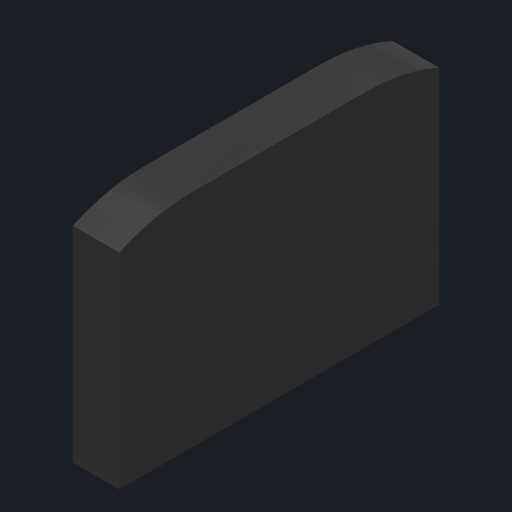
# Autodesk Inventor part: CARCASA_PANTALLA
Saved by Autodesk Inventor 2024.3 (Build 283343000, 343)
## iProperties
Created: 2024-07-02
Part Number: CARCASA_PANTALLA
Material: Steel, Mild, Welded
Document SubType Name: Modeling
Designer: Niler
Density: 7.85 g/cm^3
Appearance: Weld - Steel Mild
Author: Niler
Autodesk Inventor part; units mm, degrees
ref_plane "YZ Plane" through (0, 0, 0) normal (1, 0, 0) x (0, 1, 0)
ref_plane "XZ Plane" through (0, 0, 0) normal (0, 1, 0) x (-1, 0, 0)
ref_plane "XY Plane" through (0, 0, 0) normal (0, 0, 1) x (1, 0, 0)
sketch "Sketch1" plane through (0, 0, 0) normal (1, 0, 0) x (0, 1, 0)
  line L0 (-190, 275) -> (190, 275)
  line L1 (190, 275) -> (190, -275)
  line L2 (190, -275) -> (-190, -275)
  line L3 (-190, -275) -> (-190, 275)
  line L4 (-190, 275) -> (190, -275) construction
  line L5 (190, 275) -> (-190, -275) construction
  point P0 (0, 0)
  dimension "d0" = 550
  dimension "d1" = 380
  constraints: 12 end point, 2 midpoint, 2 parallel, 1 horizontal, 1 perpendicular
  measures "d0" distance of L0.end L1.end
  measures "d1" distance of L1.end L2.end
extrude "Extrusion1" add sketch "Sketch1" along normal mid plane 80
sketch "Sketch2" plane through (40, 0, 0) normal (1, 0, 0) x (0, 0, -1)
  line L0 (275, -190) -> (275, 190) projected
  line L1 (275, 190) -> (-275, 190) projected
  line L2 (-275, 190) -> (-275, -190) projected
  line L3 (-275, -190) -> (275, -190) projected
  line L4 (-150, 190) -> (150, 190)
  line L5 (0, 0) -> (0, 117.6253)
  arc A0 (-150, 190) -> (-275, 162.7178) centre (-150, -110) ccw
  arc A1 (275, 162.7178) -> (150, 190) centre (150, -110) ccw
  point P0 (0, 190)
  point P1 (275, 162.7178)
  dimension "d4" = 300
  dimension "d5" = 300
  constraints: 4 end point, 4 point on circle, 3 point on line, 2 centre point, 2 symmetric about line, 2 vertical alignment, 1 midpoint, 1 vertical, 1 other
  measures "d4" distance of L4.start L4.end
  measures "d5" radius of A0
extrude "Extrusion2" cut sketch "Sketch2" against normal through all contours A1 L1 L0 | L2 L1 A0
body "Solid1"
